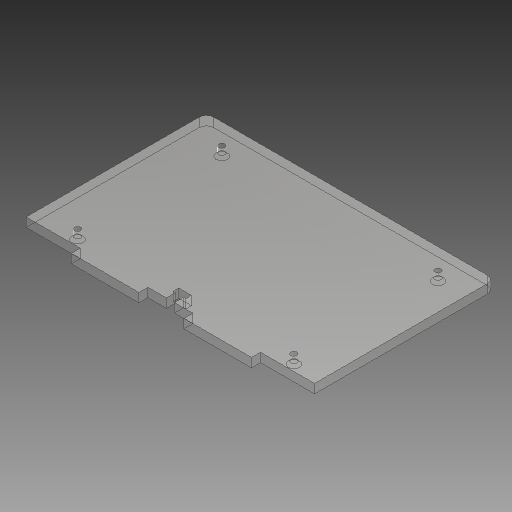
# Autodesk Inventor part: LogicHolder
Saved by Autodesk Inventor 2019 (Build 230136000, 136)
## iProperties
Created: 2018-05-15
Part Number: LogicHolder
Material: Polycarbonate, Clear
Document SubType Name: Modeling
Designer: Phil Erle
Density: 1.2 g/cm^3
Appearance: Polycarbonate - Clear
Author: Phil Erle
Autodesk Inventor part; units mm, degrees
ref_plane "YZ Plane" through (0, 0, 0) normal (1, 0, 0) x (0, 1, 0)
ref_plane "XZ Plane" through (0, 0, 0) normal (0, 1, 0) x (-1, 0, 0)
ref_plane "XY Plane" through (0, 0, 0) normal (0, 0, 1) x (1, 0, 0)
sketch "Sketch1" plane through (0, 0, 0) normal (0, 0, 1) x (1, 0, 0)
  line L0 (-80, 105) -> (80, 105)
  line L1 (80, 105) -> (80, 5)
  line L2 (80, 5) -> (50, 5)
  line L3 (50, 5) -> (50, 0)
  line L4 (-50, 0) -> (-50, 5)
  line L5 (-50, 5) -> (-80, 5)
  line L6 (-80, 105) -> (-80, 5)
  line L7 (50, 0) -> (12.5, 0)
  line L8 (12.5, 0) -> (12.5, 5)
  line L9 (12.5, 5) -> (-12.5, 5)
  line L10 (-12.5, 5) -> (-12.5, 0)
  line L11 (-12.5, 0) -> (-50, 0)
  point P0 (0, 0)
  point P1 (0, 105)
  point P2 (0, 0)
  point P3 (0, 5)
  dimension "d0" = 5
  dimension "d1" = 100
  dimension "d2" = 160
  dimension "d3" = 100
  dimension "d22" = 5
  dimension "d23" = 25
  dimension "d24" = 5
  dimension "d25" = 30
  constraints: 24 end point, 7 perpendicular, 3 point on line, 2 horizontal, 2 midpoint, 2 vertical alignment, 1 coincident, 1 horizontal alignment, 1 vertical
  measures "d0" distance of L4.start L4.end
  measures "d1" distance of L3.end L4.start
  measures "d2" distance of L0.start L0.end
  measures "d3" distance of L0.end L1.end
  measures "d22" distance of L9.end L10.end
  measures "d23" distance of L8.end L9.end
  measures "d24" distance of L2.end L3.end
  measures "d25" distance of L1.end L2.end
extrude "Extrusion1" add sketch "Sketch1" along normal blind 5
sketch "Sketch3" plane through (0, 0, 0) normal (0, 0, -1) x (-1, 0, 0)
  line L0 (60, 13.5) -> (-60, 13.5) construction
  line L1 (-60, 13.5) -> (-60, 93.5) construction
  line L2 (-60, 93.5) -> (60, 93.5) construction
  line L3 (60, 93.5) -> (60, 13.5) construction
  line L4 (60, 13.5) -> (-60, 93.5) construction
  line L5 (-60, 13.5) -> (60, 93.5) construction
  line L6 (80, 5) -> (50, 5) projected
  point P0 (0, 0)
  point P1 (60, 93.5)
  point P2 (0, 53.5)
  point P3 (0, 93.5)
  dimension "d32" = 120
  dimension "d33" = 8.5
  dimension "d34" = 80
  constraints: 12 end point, 3 coincident, 3 midpoint, 2 parallel, 1 horizontal, 1 perpendicular, 1 vertical alignment
  measures "d32" distance of L1.end L2.end
  measures "d33" distance between parallel lines of L6 L0
  measures "d34" distance of L2.end L0.start
hole "Hole1" at (60, 93.5, 0) at (-60, 93.5, 0) at (60, 13.5, 0) at (-60, 13.5, 0) direction (0, 0, 1) diameter 3.4 depth 8 tip angle 118 countersink diameter 6.3 countersink angle 90 clearance for "Countersunk Flat Head Screw DIN EN ISO 2009" size "M3" standard "DIN"
fillet "Fillet1" radius 4 2 edges at (80, 105, 2.5) (-80, 105, 2.5)
sketch "Sketch5" plane through (0, 0, 0) normal (0, 0, -1) x (-1, 0, 0)
  line L0 (-2.25, 5) -> (-2.25, 10)
  line L1 (-2.25, 10) -> (-3.5, 10)
  line L2 (-3.5, 10) -> (-3.5, 13.2)
  line L3 (-3.5, 13.2) -> (3.5, 13.2)
  line L4 (3.5, 13.2) -> (3.5, 10)
  line L5 (3.5, 10) -> (2.25, 10)
  line L6 (2.25, 10) -> (2.25, 5)
  line L7 (-12.5, 5) -> (12.5, 5) projected
  line L8 (-2.25, 5) -> (2.25, 5)
  point P0 (0, 0)
  point P1 (0, 13.2)
  point P2 (0, 5)
  point P3 (0, 5)
  dimension "d26" = 7
  dimension "d27" = 3.2
  dimension "d28" = 5
  dimension "d29" = 4.5
  constraints: 16 end point, 4 perpendicular, 3 midpoint, 3 point on line, 2 vertical alignment, 1 collinear, 1 horizontal, 1 vertical
  measures "d26" distance of L2.end L3.end
  measures "d27" distance of L1.end L2.end
  measures "d28" distance of L0.start L0.end
  measures "d29" distance between parallel lines of L6 L0
extrude "Extrusion3" cut sketch "Sketch5" against normal blind 5
equation "\"d25\" = -0.5 * d1 + 0.5 * d2"
body "Solid1"
